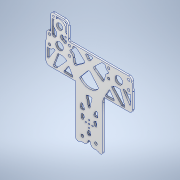
# Autodesk Inventor part: MainHolder2
Saved by Autodesk Inventor 2020.2 (Build 242310000, 310)
## iProperties
Created: 2020-01-20
Part Number: MainHolder2
Material: Aluminum 6061
Document SubType Name: Sheet Metal
Designer: Paul Lefeuvre
Density: 2.7 g/cm^3
Sheet Metal Rule: Default_mm
Appearance: Aluminum - Flat
Mass: 364.712 g
Surface Area: 716.863 cm^2
Volume: 135.078 cm^3
Author: Paul Lefeuvre
Autodesk Inventor part; units mm, degrees
ref_plane "YZ Plane" through (0, 0, 0) normal (1, 0, 0) x (0, 1, 0)
ref_plane "XZ Plane" through (0, 0, 0) normal (0, 1, 0) x (-1, 0, 0)
ref_plane "XY Plane" through (0, 0, 0) normal (0, 0, 1) x (1, 0, 0)
sketch "Sketch1" plane through (0, 0, 0) normal (0, 0, 1) x (1, 0, 0)
  circle A0 centre (-87.5, 65.6375) radius 20.6375 construction
  circle A1 centre (-116.941, 81.775) radius 3 construction
  circle A2 centre (-116.941, 81.775) radius 9.5
  circle A3 centre (-116.941, 55.5) radius 3 construction
  circle A4 centre (-116.941, 55.5) radius 9.5 construction
  circle A5 centre (-116.941, 55.5) radius 10.5 construction
  line L0 (-126.441, 81.775) -> (-126.441, 0)
  circle A6 centre (-116.941, 81.775) radius 3.6
  circle A7 centre (-116.941, 55.5) radius 3.6
  line L1 (-87.5, 45) -> (-73.2807, 45) construction
  line L2 (-116.941, 91.275) -> (0, 91.275)
  circle A8 centre (-58.059, 81.775) radius 3 construction
  circle A9 centre (-58.059, 81.775) radius 9.5 construction
  circle A10 centre (-58.059, 81.775) radius 3.6
  circle A11 centre (-58.059, 55.5) radius 3 construction
  circle A12 centre (-58.059, 55.5) radius 9.5 construction
  circle A13 centre (-58.059, 55.5) radius 10.5 construction
  circle A14 centre (-58.059, 55.5) radius 3.6
  line L3 (-48.559, 91.275) -> (-48.559, 23.4835) construction
  line L4 (0, 0) -> (0, 123.2916) construction
  line L5 (126.441, 0) -> (40, 0)
  circle A15 centre (-87.5, 65.6375) radius 10.5 construction
  circle A16 centre (-87.5, 65.6375) radius 11.1
  circle A17 centre (87.5, 65.6375) radius 20.6375 construction
  circle A18 centre (116.941, 81.775) radius 3 construction
  circle A19 centre (116.941, 81.775) radius 9.5
  circle A20 centre (116.941, 55.5) radius 3 construction
  circle A21 centre (116.941, 55.5) radius 9.5 construction
  circle A22 centre (116.941, 55.5) radius 10.5 construction
  line L6 (126.441, 81.775) -> (126.441, 0)
  circle A23 centre (116.941, 81.775) radius 3.6
  circle A24 centre (116.941, 55.5) radius 3.6
  line L7 (87.5, 45) -> (73.2807, 45) construction
  line L8 (116.941, 91.275) -> (0, 91.275)
  circle A25 centre (58.059, 81.775) radius 3 construction
  circle A26 centre (58.059, 81.775) radius 9.5 construction
  circle A27 centre (58.059, 81.775) radius 3.6
  circle A28 centre (58.059, 55.5) radius 3 construction
  circle A29 centre (58.059, 55.5) radius 9.5 construction
  circle A30 centre (58.059, 55.5) radius 10.5 construction
  circle A31 centre (58.059, 55.5) radius 3.6
  line L9 (48.559, 91.275) -> (48.559, 23.4835) construction
  arc A32 (126.441, 0) -> (126.441, 0) centre (124.441, 0) ccw
  circle A33 centre (87.5, 65.6375) radius 10.5 construction
  circle A34 centre (87.5, 65.6375) radius 11.1
  line L10 (-87.5, 122.9698) -> (-81.15, 119.3037) construction
  line L11 (-81.15, 119.3037) -> (-81.15, 111.9713) construction
  line L12 (-81.15, 111.9713) -> (-87.5, 108.3052) construction
  line L13 (-87.5, 108.3052) -> (-93.85, 111.9713) construction
  line L14 (-93.85, 111.9713) -> (-93.85, 119.3037) construction
  line L15 (-93.85, 119.3037) -> (-87.5, 122.9698) construction
  line L16 (-87.5, 65.6375) -> (-87.5, 142.8029) construction
  line L17 (-108.5, 94.6375) -> (-66.5, 94.6375) construction
  line L18 (-66.5, 94.6375) -> (-66.5, 136.6375) construction
  line L19 (-66.5, 136.6375) -> (-108.5, 136.6375) construction
  line L20 (-108.5, 136.6375) -> (-108.5, 94.6375) construction
  line L21 (-108.5, 94.6375) -> (-66.5, 136.6375) construction
  line L22 (-66.5, 94.6375) -> (-108.5, 136.6375) construction
  circle A35 centre (-105.5, 133.6375) radius 2.5
  circle A36 centre (-69.5, 97.6375) radius 2.5
  circle A37 centre (-87.5, 115.6375) radius 9
  line L23 (-113.5, 91.275) -> (-113.5, 139.6375)
  line L24 (-111.5, 141.6375) -> (-63.5, 141.6375)
  line L25 (-61.5, 139.6375) -> (-61.5, 91.275)
  arc A38 (-111.5, 141.6375) -> (-113.5, 139.6375) centre (-111.5, 139.6375) ccw
  arc A39 (-61.5, 139.6375) -> (-63.5, 141.6375) centre (-63.5, 139.6375) ccw
  line L26 (-40, 0) -> (-40, -150)
  line L27 (-40, -150) -> (40, -150)
  line L28 (40, -150) -> (40, 0)
  line L29 (-126.441, 0) -> (-40, 0)
  circle A40 centre (-20, -130) radius 4
  circle A41 centre (20, -130) radius 4
  circle A42 centre (0, -80) radius 2.1
  circle A43 centre (10, -90) radius 2.1
  circle A44 centre (-10, -90) radius 2.1
  circle A45 centre (0, -100) radius 2.1
  circle A46 centre (0, -90) radius 2.1
  line L30 (-10, -90) -> (10, -90) construction
  line L31 (0, -80) -> (0, -100) construction
  line L32 (0, -80) -> (-10, -90) construction
  line L33 (-10, -90) -> (0, -100) construction
  line L34 (0, -100) -> (10, -90) construction
  line L35 (10, -90) -> (0, -80) construction
  line L36 (-25, -115) -> (25, -115) construction
  line L37 (25, -115) -> (25, -65) construction
  line L38 (25, -65) -> (-25, -65) construction
  line L39 (-25, -65) -> (-25, -115) construction
  line L40 (-25, -115) -> (25, -65) construction
  line L41 (25, -115) -> (-25, -65) construction
  point P0 (-61.5, 91.275)
  point P1 (-40, -150)
  point P2 (40, -150)
  point P3 (40, 0)
  point P4 (126.441, 0)
  dimension "d0" = 41.275
  dimension "d1" = 6
  dimension "d2" = 19
  dimension "d3" = 6
  dimension "d4" = 19
  dimension "d5" = 21
  dimension "d6" = 0.6
  dimension "d7" = 0.6
  dimension "d8" = 6
  dimension "d9" = 19
  dimension "d10" = 0.6
  dimension "d11" = 6
  dimension "d12" = 19
  dimension "d13" = 21
  dimension "d14" = 0.6
  dimension "d15" = 25.6375
  dimension "d18" = 65.6375
  dimension "d26" = 21
  dimension "d27" = 0.6
  dimension "d80" = 12.7
  dimension "d81" = 42
  dimension "d82" = 42
  dimension "d83" = 5
  dimension "d84" = 3
  dimension "d85" = 3
  dimension "d86" = 5
  dimension "d87" = 3
  dimension "d88" = 3
  dimension "d89" = 50
  dimension "d90" = 18
  dimension "d91" = 5
  dimension "d92" = 5
  dimension "d93" = 5
  dimension "d94" = 2
  dimension "d95" = 80
  dimension "d96" = 150
  dimension "d99" = 8
  dimension "d100" = 8
  dimension "d101" = 20
  dimension "d102" = 20
  dimension "d103" = 20
  dimension "d104" = 20
  dimension "d105" = 175
  dimension "d160" = 4.2
  dimension "d161" = 4.2
  dimension "d162" = 4.2
  dimension "d163" = 4.2
  dimension "d164" = 4.2
  dimension "d165" = 20
  dimension "d166" = 20
  dimension "d167" = 50
  dimension "d168" = 50
  dimension "d170" = 15
  constraints: 84 end point, 45 centre point, 20 symmetric about line, 16 coincident, 13 point on line, 12 tangent, 10 point on circle, 8 horizontal, 8 perpendicular, 8 vertical, 6 midpoint, 4 parallel, 2 vertical alignment, 1 collinear, 1 equal radius, 36 other
  measures "d1" diameter of A1
  measures "d2" diameter of A2
  measures "d3" diameter of A3
  measures "d4" diameter of A4
  measures "d5" diameter of A5
  measures "d6" radial gap between concentric circles of A1 A6
  measures "d7" radial gap between concentric circles of A3 A7
  measures "d8" diameter of A8
  measures "d9" diameter of A9
  measures "d10" radial gap between concentric circles of A8 A10
  measures "d11" diameter of A11
  measures "d12" diameter of A12
  measures "d13" diameter of A13
  measures "d14" radial gap between concentric circles of A11 A14
  measures "d15" distance from line of L2 point (-87.5, 65.637)
  measures "d18" distance from line of L5 point (-87.5, 65.637)
  measures "d26" diameter of A15
  measures "d27" radial gap between concentric circles of A15 A16
  measures "d80" distance of L14.end L10.end
  measures "d81" distance of L19.end L18.end
  measures "d82" distance of L18.end L17.end
  measures "d83" diameter of A35
  measures "d84" distance from line of L19 A35.centre
  measures "d85" distance from line of L20 A35.centre
  measures "d86" diameter of A36
  measures "d87" distance from line of L18 A36.centre
  measures "d88" distance from line of L17 A36.centre
  measures "d89" distance of point (-87.5, 65.637) point (-87.5, 115.637)
  measures "d90" diameter of A37
  measures "d91" distance between parallel lines of L20 L23
  measures "d92" distance between parallel lines of L18 L25
  measures "d93" distance between parallel lines of L24 L19
  measures "d94" radius of A38
  measures "d95" distance of point (-40, -150) point (40, -150)
  measures "d96" distance of point (40, -150) point (40, 0)
  measures "d99" diameter of A40
  measures "d100" diameter of A41
  measures "d101" distance from line of L26 A40.centre
  measures "d102" distance from line of L28 A41.centre
  measures "d103" distance from line of L27 A41.centre
  measures "d104" distance from line of L27 A40.centre
  measures "d105" distance of A33.centre L16.start
  measures "d160" diameter of A42
  measures "d161" diameter of A43
  measures "d162" diameter of A44
  measures "d163" diameter of A45
  measures "d164" diameter of A46
  measures "d165" distance of L30.start L30.end
  measures "d166" distance of L31.start L31.end
  measures "d167" distance of L38.end L37.end
  measures "d168" distance of L37.end L36.end
  measures "d170" distance from line of A40.centre L36
extrude "Extrusion1" add sketch "Sketch1" along normal blind 5 contours A2 | A2 L2 L8 A19 L6 A32 L5 L28 L27 L26 L29 L0 | L23 A38 L24 A39 L25 L2 | A19 | L5 A32 picked at (124.8197, 0.5487)
sketch "Sketch4" plane through (0, 0, 5) normal (0, 0, 1) x (1, 0, 0)
  arc A0 (-80.4208, 98.0056) -> (-80.2388, 85.3422) centre (-77.8927, 91.7089) ccw
  arc A1 (-77.3884, 96.3059) -> (-80.4208, 98.0056) centre (-79.5892, 95.9343) ccw
  arc A2 (-17.7211, -87.7571) -> (-23.1644, -42.6162) centre (-50.7944, -68.8466) ccw
  arc A3 (-23.1644, -42.6162) -> (-23.4676, -112.946) centre (157.1876, -78.5591) ccw
  arc A4 (-17.7211, -87.7571) -> (-23.4676, -112.946) centre (20.837, -109.8036) ccw
  line L0 (-43.5068, 41.7749) -> (-43.2884, 41.3925)
  arc A5 (-26.9197, 13.3278) -> (0, 0) centre (0, 33.8505) ccw
  line L1 (-40, -16.4906) -> (-40, -150)
  line L2 (-40, -150) -> (0, -150)
  arc A6 (0, -17.7014) -> (-9.2, -20.4437) centre (0, -34.5052) ccw
  arc A7 (-2.4446, -53.1191) -> (-9.2, -20.4437) centre (-106.1207, -57.5171) ccw
  arc A8 (0, -57.8782) -> (-2.4446, -53.1191) centre (-6.6738, -58.299) ccw
  line L3 (0, 135.5567) -> (0, -151.1393) construction
  circle A9 centre (-58.059, 55.5) radius 11
  circle A10 centre (-58.059, 81.775) radius 9.5
  arc A11 (-54.5373, 72.9519) -> (-54.395, 65.8718) centre (-53.135, 69.4386) ccw
  arc A12 (-43.917, 86.275) -> (-48.5594, 81.6792) centre (-43.917, 81.6323) ccw
  arc A13 (-91.694, 45.0606) -> (-101.5959, 50.0713) centre (-87.5, 65.6375) ccw
  circle A14 centre (-116.941, 81.775) radius 9.5
  circle A15 centre (-116.941, 55.5) radius 11
  arc A16 (-101.1907, 49.5612) -> (-108.717, 48.1948) centre (-104.0824, 44.0779) ccw
  arc A17 (-107.8558, 84.5512) -> (-100.4116, 82.1992) centre (-103.3246, 85.9358) ccw
  arc A18 (-67.3546, 39.5889) -> (-84.4937, 44.8538) centre (-81.4914, 24.098) ccw
  arc A19 (-40, -16.4906) -> (-43.4158, -1.1514) centre (-76.15, -16.4906) ccw
  arc A20 (-123.0348, 64.6579) -> (-122.7168, 74.2324) centre (-126.2958, 69.5587) ccw
  circle A21 centre (-87.5, 115.6375) radius 19
  circle A22 centre (-105.5, 133.6375) radius 8
  circle A23 centre (-69.5, 97.6375) radius 8
  arc A24 (-99.9498, 82.5491) -> (-99.5, 100.9066) centre (-106.8352, 91.9021) ccw
  arc A25 (-68.7621, 112.4922) -> (-65.1691, 104.3638) centre (-60.7962, 111.1551) ccw
  line L4 (-58.059, 91.275) -> (112.2946, 91.275)
  circle A26 centre (116.941, 81.775) radius 9.5
  circle A27 centre (116.941, 55.5) radius 11
  arc A28 (101.5959, 50.0713) -> (91.694, 45.0606) centre (87.5, 65.6375) ccw
  circle A29 centre (58.059, 81.775) radius 9.5
  circle A30 centre (58.059, 55.5) radius 11
  circle A31 centre (-87.5, 115.6375) radius 9 projected
  circle A32 centre (-105.5, 133.6375) radius 2.5 projected
  circle A33 centre (-69.5, 97.6375) radius 2.5 projected
  circle A34 centre (-58.059, 81.775) radius 3.6 projected
  circle A35 centre (-87.5, 65.6375) radius 11.1 projected
  circle A36 centre (-116.941, 81.775) radius 3.6 projected
  circle A37 centre (-116.941, 55.5) radius 3.6 projected
  circle A38 centre (-58.059, 55.5) radius 3.6 projected
  circle A39 centre (116.941, 81.775) radius 3.6 projected
  circle A40 centre (87.5, 65.6375) radius 11.1 projected
  circle A41 centre (58.059, 81.775) radius 3.6 projected
  circle A42 centre (58.059, 55.5) radius 3.6 projected
  circle A43 centre (116.941, 55.5) radius 3.6 projected
  arc A44 (-47.0594, 55.4026) -> (-43.5068, 41.7749) centre (-20.0624, 55.1635) ccw
  arc A45 (-73.6062, 81.3844) -> (-67.3971, 83.5214) centre (-71.1083, 84.2155) ccw
  arc A46 (-66.5558, 86.024) -> (-68.9698, 89.6551) centre (-68.8032, 87.1479) ccw
  arc A47 (-66.6574, 68.2041) -> (-60.5525, 69.7787) centre (-63.5022, 68.5927) ccw
  arc A48 (-60.5525, 69.7787) -> (-69.6119, 76.6382) centre (-70.7985, 65.659) ccw
  line L5 (-61.5, 91.275) -> (-61.5, 139.6375) projected
  line L6 (116.941, 91.275) -> (-61.5, 91.275) projected
  arc A49 (-61.7025, 95.8489) -> (-58.059, 91.275) centre (-58.059, 95.0132) ccw
  line L7 (-113.5, 139.6375) -> (-113.5, 91.275) projected
  line L8 (-113.5, 133.6375) -> (-113.5, 90.6299)
  line L9 (-108.5, 126.2213) -> (-108.5, 86.1338)
  arc A50 (-116.941, 91.275) -> (-126.441, 81.775) centre (-116.941, 81.775) ccw projected
  line L10 (-126.4255, 82.3173) -> (-127.9231, 56.128)
  line L11 (-108.5, 94.6375) -> (-66.5, 94.6375) construction
  line L12 (-66.5, 94.6375) -> (-66.5, 136.6375) construction
  line L13 (-66.5, 136.6375) -> (-108.5, 136.6375) construction
  line L14 (-108.5, 94.6375) -> (-66.5, 136.6375) construction
  line L15 (-66.5, 94.6375) -> (-108.5, 136.6375) construction
  line L16 (-63.5, 141.6375) -> (-111.5, 141.6375) projected
  line L17 (-105.5, 141.6375) -> (-73.5, 141.6375)
  line L18 (-61.5, 129.6375) -> (-61.5, 97.6375)
  arc A51 (-61.5, 129.6375) -> (-73.5, 141.6375) centre (-73.5, 129.6375) ccw
  line L19 (-98.0838, 136.6375) -> (-73.5, 136.6375)
  arc A52 (-66.5, 129.6375) -> (-73.5, 136.6375) centre (-73.5, 129.6375) ccw
  line L20 (-66.5, 129.6375) -> (-66.5, 105.4358)
  line L21 (-126.441, 0) -> (-40, 0) projected
  line L22 (-40, 0) -> (-40, -150) projected
  arc A53 (-16.879, -146.3836) -> (-29.4222, -148.8791) centre (-20.0688, -163.1213) ccw
  arc A54 (-40, -143.1709) -> (-29.4222, -148.8791) centre (-33.1709, -143.1709) ccw
  arc A55 (0, -130.7689) -> (-3.6128, -136.7168) centre (4.8033, -137.7576) ccw
  arc A56 (-16.879, -146.3836) -> (-3.6128, -136.7168) centre (-14.7737, -135.3365) ccw
  line L23 (-40, -150) -> (40, -150) projected
  arc A57 (23.1644, -42.6162) -> (17.7211, -87.7571) centre (50.7944, -68.8466) ccw
  arc A58 (23.4676, -112.946) -> (23.1644, -42.6162) centre (-157.1876, -78.5591) ccw
  arc A59 (23.4676, -112.946) -> (17.7211, -87.7571) centre (-20.837, -109.8036) ccw
  line L24 (43.5068, 41.7749) -> (43.2884, 41.3925)
  arc A60 (0, 0) -> (26.9197, 13.3278) centre (0, 33.8505) ccw
  line L25 (58.7216, 26.363) -> (48.4214, 7.9775)
  line L26 (40, -150) -> (0, -150)
  arc A61 (9.2, -20.4437) -> (0, -17.7014) centre (0, -34.5052) ccw
  arc A62 (9.2, -20.4437) -> (2.4446, -53.1191) centre (106.1207, -57.5171) ccw
  arc A63 (2.4446, -53.1191) -> (0, -57.8782) centre (6.6738, -58.299) ccw
  arc A64 (54.395, 65.8718) -> (54.5373, 72.9519) centre (53.135, 69.4386) ccw
  arc A65 (48.5594, 81.6792) -> (43.917, 86.275) centre (43.917, 81.6323) ccw
  arc A66 (108.717, 48.1948) -> (101.1907, 49.5612) centre (104.0824, 44.0779) ccw
  arc A67 (100.4116, 82.1992) -> (107.8558, 84.5512) centre (103.3246, 85.9358) ccw
  arc A68 (84.4937, 44.8538) -> (67.3546, 39.5889) centre (81.4914, 24.098) ccw
  arc A69 (43.4158, -1.1514) -> (40, -16.4906) centre (76.15, -16.4906) ccw
  arc A70 (122.7168, 74.2324) -> (123.0348, 64.6579) centre (126.2958, 69.5587) ccw
  arc A71 (43.5068, 41.7749) -> (47.0594, 55.4026) centre (20.0624, 55.1635) ccw
  arc A72 (67.3971, 83.5214) -> (73.6062, 81.3844) centre (71.1083, 84.2155) ccw
  arc A73 (60.5525, 69.7787) -> (66.6574, 68.2041) centre (63.5022, 68.5927) ccw
  arc A74 (69.6119, 76.6382) -> (60.5525, 69.7787) centre (70.7985, 65.659) ccw
  line L27 (126.4255, 82.3173) -> (127.9231, 56.128)
  line L28 (40, -16.4906) -> (40, -150)
  arc A75 (29.4222, -148.8791) -> (16.879, -146.3836) centre (20.0688, -163.1213) ccw
  arc A76 (29.4222, -148.8791) -> (40, -143.1709) centre (33.1709, -143.1709) ccw
  arc A77 (3.6128, -136.7168) -> (0, -130.7689) centre (-4.8033, -137.7576) ccw
  arc A78 (3.6128, -136.7168) -> (16.879, -146.3836) centre (14.7737, -135.3365) ccw
  line L29 (66.4256, 86.275) -> (83.615, 86.275)
  line L30 (91.385, 86.275) -> (108.5744, 86.275)
  line L31 (-121.9113, 73.6789) -> (-122.4049, 65.047)
  line L32 (121.9113, 73.6789) -> (122.4049, 65.047)
  line L33 (-38.9167, 40.4556) -> (-15.5926, 57.4499)
  line L34 (4.1114, 74.0267) -> (9.3304, 81.5678)
  line L35 (38.9167, 40.4556) -> (15.5926, 57.4499)
  line L36 (-4.1114, 74.0267) -> (-9.3304, 81.5678)
  line L37 (-26.8236, 17.085) -> (-3.8161, 44.2617)
  line L38 (15.134, 65.1543) -> (37.0068, 85.473)
  line L39 (26.8236, 17.085) -> (3.8161, 44.2617)
  line L40 (-15.134, 65.1543) -> (-37.0068, 85.473)
  arc A79 (-15.5926, 57.4499) -> (-15.134, 65.1543) centre (-18.537, 61.491) ccw
  arc A80 (-4.1114, 74.0267) -> (4.1114, 74.0267) centre (0, 76.8721) ccw
  arc A81 (15.134, 65.1543) -> (15.5926, 57.4499) centre (18.537, 61.491) ccw
  arc A82 (3.8161, 44.2617) -> (-3.8161, 44.2617) centre (0, 41.031) ccw
  line L41 (0, 86.275) -> (-6.8635, 86.275)
  line L42 (-39.0486, 86.275) -> (-43.917, 86.275)
  line L43 (0, 86.275) -> (6.8635, 86.275)
  line L44 (39.0486, 86.275) -> (43.917, 86.275)
  arc A83 (-43.2884, 41.3925) -> (-38.9167, 40.4556) centre (-40.6833, 42.8802) ccw
  arc A84 (-26.8236, 17.085) -> (-26.9197, 13.3278) centre (-24.534, 15.1466) ccw
  arc A85 (26.9197, 13.3278) -> (26.8236, 17.085) centre (24.534, 15.1466) ccw
  arc A86 (38.9167, 40.4556) -> (43.2884, 41.3925) centre (40.6833, 42.8802) ccw
  arc A87 (39.0486, 86.275) -> (37.0068, 85.473) centre (39.0486, 83.275) ccw
  arc A88 (9.3304, 81.5678) -> (6.8635, 86.275) centre (6.8635, 83.275) ccw
  arc A89 (-6.8635, 86.275) -> (-9.3304, 81.5678) centre (-6.8635, 83.275) ccw
  arc A90 (-37.0068, 85.473) -> (-39.0486, 86.275) centre (-39.0486, 83.275) ccw
  line L45 (-127.941, 55.5) -> (-127.941, 10)
  line L46 (-117.941, 0) -> (-45.2268, 0)
  arc A91 (-127.941, 10) -> (-117.941, 0) centre (-117.941, 10) ccw
  line L47 (-122.941, 20.5481) -> (-122.941, 46.2805)
  line L48 (-95.9059, 5.6446) -> (-67.2321, 36.7561)
  line L49 (-74.3423, 8.1067) -> (-62.1325, 26.4919)
  line L50 (-101.2554, 47.5083) -> (-119.258, 19.4676)
  line L51 (127.941, 55.5) -> (127.941, 10)
  line L52 (117.941, 0) -> (45.2268, 0)
  arc A92 (117.941, 0) -> (127.941, 10) centre (117.941, 10) ccw
  line L53 (122.941, 20.5481) -> (122.941, 46.2805)
  line L54 (95.9059, 5.6446) -> (67.2321, 36.7561)
  line L55 (73.6986, 9.076) -> (62.1325, 26.4919)
  line L56 (101.2554, 47.5083) -> (119.258, 19.4676)
  line L57 (-50.2548, 5.002) -> (-73.2836, 6.023)
  line L58 (-97.3766, 5) -> (-103.9267, 5)
  arc A93 (-122.941, 20.5481) -> (-119.258, 19.4676) centre (-120.941, 20.5481) ccw
  arc A94 (-105.8589, 7.5163) -> (-103.9267, 5) centre (-103.9267, 7) ccw
  arc A95 (-97.3766, 5) -> (-95.9059, 5.6446) centre (-97.3766, 7) ccw
  arc A96 (-67.2321, 36.7561) -> (-67.3546, 39.5889) centre (-68.7028, 38.1116) ccw
  arc A97 (-58.7216, 26.363) -> (-62.1325, 26.4919) centre (-60.4665, 25.3855) ccw
  arc A98 (-74.3423, 8.1067) -> (-73.2836, 6.023) centre (-73.2241, 7.3641) ccw
  arc A99 (-101.2554, 47.5083) -> (-101.5959, 50.0713) centre (-102.9384, 48.5888) ccw
  line L59 (-58.7216, 26.363) -> (-48.4214, 7.9775)
  line L60 (-44.6121, 1.1781) -> (-43.9521, 0)
  arc A100 (-50.2548, 5.002) -> (-48.4214, 7.9775) centre (-50.1662, 7) ccw
  arc A101 (-43.4158, -1.1514) -> (-45.2268, 0) centre (-45.2268, -2) ccw
  line L61 (50.2548, 5.002) -> (72.1211, 5.9715)
  line L62 (97.3766, 5) -> (103.9292, 5)
  arc A102 (62.1325, 26.4919) -> (58.7216, 26.363) centre (60.4665, 25.3855) ccw
  arc A103 (48.4214, 7.9775) -> (50.2548, 5.002) centre (50.1662, 7) ccw
  arc A104 (72.1211, 5.9715) -> (73.6986, 9.076) centre (72.0325, 7.9695) ccw
  arc A105 (95.9059, 5.6446) -> (97.3766, 5) centre (97.3766, 7) ccw
  arc A106 (103.9292, 5) -> (105.867, 7.4948) centre (103.9292, 7) ccw
  arc A107 (67.3546, 39.5889) -> (67.2321, 36.7561) centre (68.7028, 38.1116) ccw
  arc A108 (119.258, 19.4676) -> (122.941, 20.5481) centre (120.941, 20.5481) ccw
  arc A109 (101.5959, 50.0713) -> (101.2554, 47.5083) centre (102.9384, 48.5888) ccw
  arc A110 (45.2268, 0) -> (43.4158, -1.1514) centre (45.2268, -2) ccw
  circle A111 centre (-20, -130) radius 4
  circle A112 centre (20, -130) radius 4
  circle A113 centre (20, -130) radius 4 projected
  circle A114 centre (-20, -130) radius 4 projected
  line L63 (-126.441, 4.7322) -> (-126.441, 0)
  line L64 (126.4255, 0) -> (117.941, 0)
  line L65 (40, 0) -> (126.441, 0) projected
  line L66 (126.441, 0) -> (126.441, 4.7322)
  line L67 (126.441, 0) -> (126.441, 81.775) projected
  line L68 (-113.5, 133.6375) -> (-113.5, 141.6375)
  line L69 (-113.5, 141.6375) -> (-105.5, 141.6375)
  line L70 (-73.5, 141.6375) -> (-61.5, 141.6375)
  line L71 (-61.5, 141.6375) -> (-61.5, 129.6375)
  line L72 (-61.5, 97.6375) -> (-61.5, 93.5526)
  line L73 (-105.8589, 7.5163) -> (-91.694, 45.0606)
  line L74 (105.867, 7.4948) -> (91.694, 45.0606)
  circle A115 centre (0, -100) radius 2.1 projected
  arc A116 (-2.5882, -105.413) -> (0, -106) centre (0, -100) ccw
  arc A117 (-5.9308, -117.4348) -> (-2.5882, -105.413) centre (-43.8339, -100.4207) ccw
  arc A118 (0, -123.9139) -> (-5.9308, -117.4348) centre (-6.5045, -123.9139) ccw
  arc A119 (0, -106) -> (2.5882, -105.413) centre (0, -100) ccw
  arc A120 (2.5882, -105.413) -> (5.9308, -117.4348) centre (43.8339, -100.4207) ccw
  arc A121 (5.9308, -117.4348) -> (0, -123.9139) centre (6.5045, -123.9139) ccw
  circle A122 centre (-10, -90) radius 2.1 projected
  circle A123 centre (0, -90) radius 2.1 projected
  circle A124 centre (0, -80) radius 2.1 projected
  circle A125 centre (10, -90) radius 2.1 projected
  point P0 (-40, -7.0543)
  point P1 (-63.1952, 34.3482)
  point P2 (-106.5313, 94.6375)
  point P3 (40, -7.0543)
  point P4 (63.1952, 34.3482)
  point P5 (12.5881, 86.275)
  point P6 (-28.3236, 15.3132)
  point P7 (37.8702, 86.275)
  point P8 (-12.5881, 86.275)
  point P9 (28.3236, 15.3132)
  point P10 (-37.8702, 86.275)
  point P11 (0, 48.7693)
  point P12 (41.626, 38.4815)
  point P13 (-41.626, 38.4815)
  point P14 (-43.9804, 0)
  point P15 (-46.6652, 4.8428)
  point P16 (-122.941, 10)
  point P17 (-96.5, 5)
  point P18 (-75.6562, 6.1283)
  point P19 (-95.5145, 46.227)
  point P20 (96.5, 5)
  point P21 (75.6562, 6.1283)
  point P22 (95.5145, 46.227)
  point P23 (100.303, 48.9917)
  point P24 (-65.9354, 38.1631)
  point P25 (-60.3216, 29.2188)
  point P26 (-106.5313, 5)
  point P27 (-122.941, 13.7311)
  point P28 (-100.303, 48.9917)
  point P29 (44.6121, 1.1781)
  point P30 (46.6652, 4.8428)
  point P31 (43.9804, 0)
  point P32 (65.9354, 38.1631)
  point P33 (60.3216, 29.2188)
  point P34 (106.5313, 5)
  point P35 (122.941, 13.7311)
  point P36 (-97.7554, 131.6321)
  point P37 (-103.4946, 125.8929)
  point P38 (-121.9217, 73.4982)
  point P39 (-122.3993, 65.1463)
  point P40 (122.3993, 65.1463)
  point P41 (121.9217, 73.4982)
  point P42 (67.3971, 83.5214)
  point P43 (73.6062, 81.3844)
  point P44 (100.4116, 82.1992)
  point P45 (108.717, 48.1948)
  point P46 (84.4937, 44.8538)
  point P47 (-33.1709, -150)
  point P48 (33.1709, -150)
  point P49 (-40, -143.1709)
  point P50 (47.0594, 55.4026)
  point P51 (48.5594, 81.6792)
  point P52 (-48.559, 81.775)
  point P53 (127.941, 55.5)
  point P54 (122.7168, 74.2324)
  point P55 (123.0348, 64.6579)
  point P56 (108.2167, 62.1997)
  point P57 (105.9414, 55.5919)
  point P58 (66.7833, 62.1997)
  point P59 (58.059, 91.275)
  point P60 (-66.7833, 62.1997)
  point P61 (-108.2167, 62.1997)
  point P62 (-105.9414, 55.5919)
  dimension "d124" = 19
  dimension "d125" = 19
  dimension "d128" = 22
  dimension "d132" = 42
  dimension "d121" = 22
  dimension "d122" = 22
  dimension "d123" = 19
  dimension "d126" = 19
  dimension "d127" = 22
  dimension "d129" = 16
  dimension "d130" = 16
  dimension "d131" = 38
  dimension "d133" = 42
  dimension "d134" = 5
  dimension "d135" = 42
  dimension "d136" = 42
  dimension "d137" = 12
  dimension "d138" = 5
  dimension "d142" = 5
  dimension "d143" = 5
  dimension "d144" = 5
  dimension "d145" = 5
  dimension "d148" = 5
  dimension "d149" = 3
  dimension "d150" = 10
  dimension "d152" = 2
  dimension "d153" = 2
  dimension "d154" = 2
  dimension "d155" = 2
  dimension "d172" = 12
  constraints: 228 point on circle, 130 end point, 107 tangent, 101 centre point, 79 horizontal alignment, 58 point on line, 45 equal radius, 14 concentric, 7 parallel, 6 horizontal, 4 coincident, 3 vertical, 2 collinear, 2 equal length, 2 midpoint, 2 perpendicular, 59 other
  measures "d121" diameter of A9
  measures "d122" diameter of A15
  measures "d123" diameter of A10
  measures "d126" diameter of A26
  measures "d127" diameter of A30
  measures "d129" diameter of A22
  measures "d130" diameter of A23
  measures "d131" diameter of A21
  measures "d133" diameter of A28
  measures "d134" distance between parallel lines of L7 L9
  measures "d135" distance of L13.end L12.end
  measures "d136" distance of L12.end L11.end
  measures "d137" radius of A51
  measures "d138" distance between parallel lines of L17 L19
  measures "d142" distance between parallel lines of L4 L29
  measures "d143" distance between parallel lines of L4 L30
  measures "d144" distance between parallel lines of L10 L31
  measures "d145" distance between parallel lines of L27 L32
  measures "d148" radius of A79
  measures "d149" radius of A83
  measures "d150" radius of A91
  measures "d152" radius of A93
  measures "d153" radius of A100
  measures "d154" radius of A102
  measures "d155" radius of A110
  measures "d172" diameter of A116
extrude "Extrusion2" cut sketch "Sketch4" against normal blind 10 contours A1 A23 A46 A10 A45 A13 A0 | A24 A13 A17 A14 L9 A22 A21 | A23 L5 A49 | A22 L19 A52 L20 A25 A21 | L7 L68 L69 L16 A22 | A10 A12 L42 A90 L40 A79 L33 A83 L0 A44 A9 A11 | A51 L16 L70 L71 L5 | A29 A64 A30 A71 L24 A86 L35 A81 L38 A87 L44 A65 | A99 L50 A93 L47 A15 A16 | A91 L21 L63 | L53 A108 L56 A109 A66 A27 | L66 L65 L64 A92 | A54 L2 L1 | A54 A53 A56 A55 A77 A78 A75 A76 L23 L2 | L28 L23 A76 | A4 A3 A2 | A84 L37 A82 L39 A85 A60 A5 | A61 A62 A63 A8 A7 A6 | A13 A18 A96 L48 A95 L58 A94 L73 | A28 L74 A106 L62 A105 L54 A107 A68 | A58 A59 A57 | A102 L55 A104 L61 A103 L25 | A80 L36 A89 L41 L43 A88 L34 | L49 A97 L59 A100 L57 A98 | A116 A119 A120 A121 A118 A117
extrude "Extrusion3" add sketch "Sketch4" against normal blind 5 contours A13 A9 A44 L0 A83 L33 A79 L40 A90 L42 A12 A10 L4 A29 A65 L44 A87 L38 A81 L35 A86 L24 A71 A30 A28 A27 A109 L56 A108 L53 L67 A92 L52 A110 A69 L28 A76 A75 A78 A77 A55 A56 A53 A54 L1 L22 L21 A91 L45 A15 L47 A93 L50 A99 | A13 A15 | A49 L6 L5 | A15 L10 A14 A20 L31 | L27 A27 L67 A26 | L67 A27 A70 L32 A26 | A27 L67 | L67 A27 A28 | L51 A92 L67 A27 picked at (-125.3269, 54.3111)
sketch "Sketch5" plane through (0, 0, 5) normal (0, 0, 1) x (1, 0, 0)
  line L0 (-25, -115) -> (25, -115) construction
  line L1 (25, -115) -> (25, -65) construction
  line L2 (25, -65) -> (-25, -65) construction
  line L3 (-25, -65) -> (-25, -115) construction
  line L4 (-25, -115) -> (25, -65) construction
  line L5 (25, -115) -> (-25, -65) construction
  circle A0 centre (0, -90) radius 2.1 projected
  arc A1 (-23.1644, -42.6162) -> (-23.4676, -112.946) centre (157.1876, -78.5591) ccw projected
  arc A2 (-17.7211, -87.7571) -> (-23.1644, -42.6162) centre (-50.7944, -68.8466) ccw projected
  arc A3 (-24.3528, -49.2021) -> (-25.6877, -59.1839) centre (157.1876, -78.5591) ccw
  line L6 (-16.9639, -62.5) -> (-22.7044, -62.5)
  line L7 (-22.5, -75.8563) -> (-22.5, -84.7376)
  line L8 (-17.3934, -73.7203) -> (-14.8932, -76.1861)
  arc A4 (-17.3934, -73.7203) -> (-22.5, -75.8563) centre (-19.5, -75.8563) ccw
  arc A5 (-25.6877, -59.1839) -> (-22.7044, -62.5) centre (-22.7044, -59.5) ccw
  arc A6 (-14.0722, -58.7011) -> (-18.8781, -48.0428) centre (-50.7944, -68.8466) ccw
  arc A7 (-16.9639, -62.5) -> (-14.0722, -58.7011) centre (-16.9639, -59.5) ccw
  arc A8 (-17.7211, -87.7571) -> (-14.1111, -79.132) centre (-50.7944, -68.8466) ccw
  arc A9 (-14.1111, -79.132) -> (-14.8932, -76.1861) centre (-16.9997, -78.3221) ccw
  arc A10 (-22.5, -84.7376) -> (-16.8251, -86.0959) centre (-19.5, -84.7376) ccw
  line L9 (0, -90) -> (0, -46.3331) construction
  arc A11 (-17.7211, -87.7571) -> (-23.4676, -112.946) centre (20.837, -109.8036) ccw projected
  arc A12 (-23.08, -103.1648) -> (-25.0597, -103.1491) centre (-24.0687, -103.0153) ccw
  arc A13 (-23.08, -103.1648) -> (-23.4676, -112.946) centre (20.837, -109.8036) ccw
  arc A14 (-25.0597, -103.1491) -> (-23.4676, -112.946) centre (157.1876, -78.5591) ccw
  arc A15 (-23.1644, -42.6162) -> (-23.4676, -112.946) centre (157.1876, -78.5591) ccw
  arc A16 (-17.7211, -87.7571) -> (-23.1644, -42.6162) centre (-50.7944, -68.8466) ccw
  arc A17 (-17.7211, -87.7571) -> (-23.4676, -112.946) centre (20.837, -109.8036) ccw
  arc A18 (-18.8781, -48.0428) -> (-24.3528, -49.2021) centre (-21.3913, -49.681) ccw
  line L10 (25, -65) -> (25, -115) construction
  arc A19 (23.4676, -112.946) -> (23.1644, -42.6162) centre (-157.1876, -78.5591) ccw
  arc A20 (23.1644, -42.6162) -> (17.7211, -87.7571) centre (50.7944, -68.8466) ccw
  arc A21 (25.6877, -59.1839) -> (24.3528, -49.2021) centre (-157.1876, -78.5591) ccw
  line L11 (16.9639, -62.5) -> (22.7044, -62.5)
  line L12 (22.5, -75.8563) -> (22.5, -84.7376)
  line L13 (17.3934, -73.7203) -> (14.8932, -76.1861)
  arc A22 (22.5, -75.8563) -> (17.3934, -73.7203) centre (19.5, -75.8563) ccw
  arc A23 (22.7044, -62.5) -> (25.6877, -59.1839) centre (22.7044, -59.5) ccw
  arc A24 (18.8781, -48.0428) -> (14.0722, -58.7011) centre (50.7944, -68.8466) ccw
  arc A25 (14.0722, -58.7011) -> (16.9639, -62.5) centre (16.9639, -59.5) ccw
  arc A26 (14.1111, -79.132) -> (17.7211, -87.7571) centre (50.7944, -68.8466) ccw
  arc A27 (14.8932, -76.1861) -> (14.1111, -79.132) centre (16.9997, -78.3221) ccw
  arc A28 (16.8251, -86.0959) -> (22.5, -84.7376) centre (19.5, -84.7376) ccw
  arc A29 (23.4676, -112.946) -> (17.7211, -87.7571) centre (-20.837, -109.8036) ccw
  arc A30 (25.0597, -103.1491) -> (23.08, -103.1648) centre (24.0687, -103.0153) ccw
  arc A31 (23.4676, -112.946) -> (23.08, -103.1648) centre (-20.837, -109.8036) ccw
  arc A32 (23.4676, -112.946) -> (25.0597, -103.1491) centre (-157.1876, -78.5591) ccw
  arc A33 (23.4676, -112.946) -> (23.1644, -42.6162) centre (-157.1876, -78.5591) ccw
  arc A34 (23.1644, -42.6162) -> (17.7211, -87.7571) centre (50.7944, -68.8466) ccw
  arc A35 (23.4676, -112.946) -> (17.7211, -87.7571) centre (-20.837, -109.8036) ccw
  arc A36 (24.3528, -49.2021) -> (18.8781, -48.0428) centre (21.3913, -49.681) ccw
  arc A37 (9.2, -20.4437) -> (-9.2, -20.4437) centre (0, -34.5052) ccw projected
  arc A38 (-2.4446, -53.1191) -> (-9.2, -20.4437) centre (-106.1207, -57.5171) ccw projected
  arc A39 (9.2, -20.4437) -> (2.4446, -53.1191) centre (106.1207, -57.5171) ccw projected
  arc A40 (2.4446, -53.1191) -> (0, -57.8782) centre (6.6738, -58.299) ccw projected
  arc A41 (0, -57.8782) -> (-2.4446, -53.1191) centre (-6.6738, -58.299) ccw projected
  arc A42 (9.2, -20.4437) -> (-9.2, -20.4437) centre (0, -34.5052) ccw projected
  arc A43 (-6.6816, -19.0869) -> (-8.3163, -22.842) centre (-5.4887, -21.8396) ccw
  arc A44 (8.3163, -22.842) -> (6.6816, -19.0869) centre (5.4887, -21.8396) ccw
  arc A45 (-2.9818, -46.0965) -> (2.9818, -46.0965) centre (0, -45.7663) ccw
  arc A46 (-5.9308, -117.4348) -> (-2.5882, -105.413) centre (-43.8339, -100.4207) ccw projected
  arc A47 (-2.5882, -105.413) -> (2.5882, -105.413) centre (0, -100) ccw projected
  arc A48 (2.5882, -105.413) -> (5.9308, -117.4348) centre (43.8339, -100.4207) ccw projected
  arc A49 (5.9308, -117.4348) -> (0, -123.9139) centre (6.5045, -123.9139) ccw projected
  arc A50 (0, -123.9139) -> (-5.9308, -117.4348) centre (-6.5045, -123.9139) ccw projected
  arc A51 (2.5882, -105.413) -> (5.9308, -117.4348) centre (43.8339, -100.4207) ccw projected
  arc A52 (3.1347, -108.7697) -> (-3.1347, -108.7697) centre (0, -109.4127) ccw
  arc A53 (3.3835, -118.2071) -> (4.7652, -114.5544) centre (1.9441, -115.575) ccw
  arc A54 (-4.7652, -114.5544) -> (-3.3835, -118.2071) centre (-1.9441, -115.575) ccw
  arc A55 (-2.0531, -119.1712) -> (2.0531, -119.1712) centre (0, -116.9838) ccw
  arc A56 (3.6128, -136.7168) -> (0, -130.7689) centre (-4.8033, -137.7576) ccw projected
  arc A57 (0, -130.7689) -> (-3.6128, -136.7168) centre (4.8033, -137.7576) ccw projected
  arc A58 (2.6294, -133.6749) -> (-2.6294, -133.6749) centre (0, -135.1192) ccw
  arc A59 (9.2, -20.4437) -> (-9.2, -20.4437) centre (0, -34.5052) ccw
  arc A60 (-2.4446, -53.1191) -> (-9.2, -20.4437) centre (-106.1207, -57.5171) ccw
  arc A61 (9.2, -20.4437) -> (2.4446, -53.1191) centre (106.1207, -57.5171) ccw
  arc A62 (2.4446, -53.1191) -> (0, -57.8782) centre (6.6738, -58.299) ccw projected
  arc A63 (2.4446, -53.1191) -> (0, -57.8782) centre (6.6738, -58.299) ccw
  arc A64 (0, -57.8782) -> (-2.4446, -53.1191) centre (-6.6738, -58.299) ccw
  arc A65 (-5.9308, -117.4348) -> (-2.5882, -105.413) centre (-43.8339, -100.4207) ccw
  arc A66 (-2.5882, -105.413) -> (2.5882, -105.413) centre (0, -100) ccw
  arc A67 (2.5882, -105.413) -> (5.9308, -117.4348) centre (43.8339, -100.4207) ccw
  arc A68 (5.9308, -117.4348) -> (0, -123.9139) centre (6.5045, -123.9139) ccw
  arc A69 (0, -123.9139) -> (-5.9308, -117.4348) centre (-6.5045, -123.9139) ccw
  arc A70 (0, -130.7689) -> (-3.6128, -136.7168) centre (4.8033, -137.7576) ccw
  arc A71 (3.6128, -136.7168) -> (0, -130.7689) centre (-4.8033, -137.7576) ccw
  point P0 (0, 0)
  point P1 (0, -90)
  point P2 (23.1644, -42.6162)
  point P3 (23.4676, -112.946)
  point P4 (-13.2288, -62.5)
  point P5 (-26.0086, -62.5)
  point P6 (-22.5, -67.5)
  point P7 (-22.5, -100.0734)
  point P8 (-13.6678, -77.3946)
  point P9 (-14.1111, -79.132)
  point P10 (-25.6877, -59.1839)
  point P11 (13.2288, -62.5)
  point P12 (26.0086, -62.5)
  point P13 (22.5, -67.5)
  point P14 (22.5, -100.0734)
  point P15 (13.6678, -77.3946)
  point P16 (-25.6877, -59.1839)
  point P17 (-14.1111, -79.132)
  point P18 (-16.8251, -86.0959)
  point P19 (-24.3528, -49.2021)
  point P20 (-18.8781, -48.0428)
  point P21 (24.3528, -49.2021)
  point P22 (25.6877, -59.1839)
  point P23 (14.1111, -79.132)
  point P24 (-6.6816, -19.0869)
  point P25 (6.6816, -19.0869)
  point P26 (0, -106)
  point P27 (1.5581, -105.7942)
  point P28 (3.1347, -108.7697)
  dimension "d173" = 50
  dimension "d174" = 50
  dimension "d177" = 2.5
  dimension "d179" = 2.5
  dimension "d183" = 3
  dimension "d184" = 3
  dimension "d191" = 1
  dimension "d196" = 3
  dimension "d197" = 3
  dimension "d199" = 3
  dimension "d200" = 3
  dimension "d201" = 3
  dimension "d202" = 3
  dimension "d204" = 3
  dimension "d205" = 3
  dimension "d206" = 3
  dimension "d207" = 3
  dimension "d209" = 3.2
  constraints: 144 point on circle, 52 centre point, 41 symmetric about line, 29 tangent, 28 end point, 16 concentric, 10 point on line, 3 midpoint, 2 horizontal, 2 parallel, 2 vertical, 1 coincident, 1 equal radius, 1 perpendicular, 29 other
  measures "d173" distance of L2.end L1.end
  measures "d174" distance of L1.end L0.end
  measures "d177" distance between parallel lines of L3 L7
  measures "d179" distance between parallel lines of L2 L6
  measures "d183" radius of A9
  measures "d184" radius of A10
  measures "d191" radius of A12
  measures "d196" radius of A5
  measures "d197" radius of A18
  measures "d199" radius of A4
  measures "d200" radius of A45
  measures "d201" radius of A44
  measures "d202" radius of A43
  measures "d204" radius of A53
  measures "d205" radius of A54
  measures "d206" radius of A55
  measures "d207" radius of A58
  measures "d209" radius of A52
extrude "Extrusion4" add sketch "Sketch5" against normal blind 5 contours A2 A18 A1 | A5 L6 A7 A2 A9 L8 A4 L7 A10 A11 A12 A1 | A12 A11 A1 | A29 A30 A19 | A30 A29 A20 A28 L12 A22 L13 A27 A25 L11 A23 A19 | A36 A20 A19 | A39 A44 A37 | A43 A38 A37 | A39 A40 A41 A38 A45 | A46 A54 A50 | A46 A47 A48 A52 | A55 A49 A50 | A48 A49 A53 | A58 A57 A56
equation "\"BendRadius\" = Thickness"
equation "\"BendReliefWidth\" = Thickness"
equation "\"BendReliefDepth\" = 0.5 * Thickness"
equation "\"CornerReliefSize\" = 4 * Thickness"
equation "\"MinimumRemnant\" = 2 * Thickness"
equation "\"TransitionRadius\" = BendRadius"
equation "\"JacobiRadiusSize\" = BendRadius"
equation "\"GapSize\" = Thickness"
equation "\"d44\" = Thickness"
equation "\"Thickness\" = 2"
body "Solid1"
